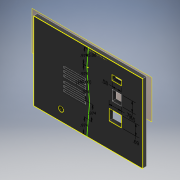
# Autodesk Inventor part: compnent box front
Saved by Autodesk Inventor 2021 (Build 250183000, 183)
## iProperties
Created: 2023-01-12
Part Number: compnent box front
Material: Generic
Document SubType Name: Modeling
Designer: boyle
Density: 1 g/cm^3
Appearance: Default
Author: boyle
Autodesk Inventor part; units mm, degrees
ref_plane "YZ Plane" through (0, 0, 0) normal (1, 0, 0) x (0, 1, 0)
ref_plane "XZ Plane" through (0, 0, 0) normal (0, 1, 0) x (-1, 0, 0)
ref_plane "XY Plane" through (0, 0, 0) normal (0, 0, 1) x (1, 0, 0)
ref_plane "Work Plane1" through (0, 0, 0) normal (0, 0, 1) x (1, 0, 0)
sketch "Sketch1" plane through (0, 0, 0) normal (0, 0, 1) x (1, 0, 0)
  line L0 (88.9, -98.425) -> (-88.9, -98.425)
  line L1 (-88.9, -98.425) -> (-88.9, -28.575)
  line L2 (-88.9, -28.575) -> (-88.9, 28.575)
  line L3 (-88.9, 28.575) -> (-85.09, 28.575)
  line L4 (88.9, 28.575) -> (88.9, -28.575)
  line L5 (85.09, 28.575) -> (88.9, 28.575)
  line L6 (88.9, -28.575) -> (88.9, -98.425)
  line L7 (-88.9, 28.575) -> (88.9, 28.575)
  line L8 (88.9, 28.575) -> (88.9, -98.425)
  line L9 (88.9, -98.425) -> (-88.9, -98.425)
  line L10 (-88.9, -98.425) -> (-88.9, 28.575)
  point P0 (0, 0)
extrude "Extrusion1" add sketch "Sketch1" along normal blind 6.35
sketch "Sketch2" plane through (0, 0, 6.35) normal (0, 0, 1) x (1, 0, 0)
  line L0 (-88.9, -98.425) -> (88.9, -98.425) projected
  line L1 (-88.9, -98.425) -> (-88.9, -28.575)
  line L2 (-88.9, 28.575) -> (-88.9, -98.425) projected
  line L3 (88.9, -98.425) -> (88.9, 28.575) projected
  circle A0 centre (-44.45, -80.9625) radius 3.937
  line L4 (-88.9, 28.575) -> (88.9, 28.575)
  line L5 (88.9, 28.575) -> (88.9, -28.575)
  line L6 (-88.9, -28.575) -> (-88.9, 28.575)
  line L7 (88.9, 28.575) -> (-88.9, 28.575) projected
  line L8 (-66.675, -80.9625) -> (-44.45, -80.9625)
  line L9 (38.7824, 9.525) -> (54.0224, 9.525)
  line L10 (54.0224, 9.525) -> (54.0224, 1.397)
  line L11 (54.0224, 1.397) -> (38.7824, 1.397)
  line L12 (38.7824, 1.397) -> (38.7824, 9.525)
  line L13 (38.7824, 9.525) -> (54.0224, 1.397) construction
  line L14 (54.0224, 9.525) -> (38.7824, 1.397) construction
  line L15 (34.2724, -40.503) -> (54.0224, -40.503)
  line L16 (54.0224, -40.503) -> (54.0224, -58.103)
  line L17 (54.0224, -58.103) -> (34.2724, -58.103)
  line L18 (34.2724, -58.103) -> (34.2724, -40.503)
  line L19 (34.2724, -40.503) -> (54.0224, -58.103) construction
  line L20 (54.0224, -40.503) -> (34.2724, -58.103) construction
  line L21 (39.3724, -11.303) -> (54.0224, -11.303)
  line L22 (54.0224, -11.303) -> (54.0224, -27.803)
  line L23 (39.3724, -27.803) -> (39.3724, -11.303)
  line L24 (39.3724, -11.303) -> (54.0224, -27.803) construction
  line L25 (54.0224, -11.303) -> (39.3724, -27.803) construction
  line L26 (-39.6628, -17.9021) -> (-3.6628, -17.9021)
  line L27 (-3.6628, -17.9021) -> (-3.6628, -53.9021)
  line L28 (-3.6628, -53.9021) -> (-39.6628, -53.9021)
  line L29 (-39.6628, -17.9021) -> (-3.6628, -53.9021) construction
  line L30 (-3.6628, -17.9021) -> (-39.6628, -53.9021) construction
  line L31 (-39.6628, -17.9021) -> (-39.6628, -53.9021)
  line L32 (-21.6628, -17.9021) -> (-21.6628, -20.9021)
  line L33 (-21.6628, -20.9021) -> (-39.6628, -20.9021)
  line L34 (-21.6628, -20.9021) -> (-3.6628, -20.9021)
  line L35 (-21.6628, -20.9021) -> (-21.6628, -23.9021)
  line L36 (-21.6628, -23.9021) -> (-39.6628, -23.9021)
  line L37 (-21.6628, -23.9021) -> (-3.6628, -23.9021)
  line L38 (-21.6628, -23.9021) -> (-21.6628, -26.9021)
  line L39 (-21.6628, -26.9021) -> (-39.6628, -26.9021)
  line L40 (-21.6628, -26.9021) -> (-3.6628, -26.9021)
  line L41 (-21.6628, -26.9021) -> (-21.6628, -29.9021)
  line L42 (-21.6628, -29.9021) -> (-39.6628, -29.9021)
  line L43 (-21.6628, -29.9021) -> (-3.6628, -29.9021)
  line L44 (-21.6628, -29.9021) -> (-21.6628, -32.9021)
  line L45 (-21.6628, -32.9021) -> (-39.6628, -32.9021)
  line L46 (-21.6628, -32.9021) -> (-3.6628, -32.9021)
  line L47 (-21.6628, -32.9021) -> (-21.6628, -35.9021)
  line L48 (-21.6628, -35.9021) -> (-39.6628, -35.9021)
  line L49 (-21.6628, -35.9021) -> (-3.6628, -35.9021)
  line L50 (-21.6628, -35.9021) -> (-21.6628, -38.9021)
  line L51 (-21.6628, -38.9021) -> (-39.6628, -38.9021)
  line L52 (-21.6628, -38.9021) -> (-3.6628, -38.9021)
  line L53 (-21.6628, -38.9021) -> (-21.6628, -41.9021)
  line L54 (-21.6628, -41.9021) -> (-39.6628, -41.9021)
  line L55 (-21.6628, -41.9021) -> (-3.6628, -41.9021)
  line L56 (-21.6628, -41.9021) -> (-21.6628, -44.9021)
  line L57 (-21.6628, -44.9021) -> (-39.6628, -44.9021)
  line L58 (-21.6628, -44.9021) -> (-3.6628, -44.9021)
  line L59 (-21.6628, -44.9021) -> (-21.6628, -47.9021)
  line L60 (-21.6628, -47.9021) -> (-39.6628, -47.9021)
  line L61 (-21.6628, -47.9021) -> (-3.6628, -47.9021)
  line L62 (-21.6628, -47.9021) -> (-21.6628, -50.9021)
  line L63 (-21.6628, -50.9021) -> (-39.6628, -50.9021)
  line L64 (-21.6628, -50.9021) -> (-3.6628, -50.9021)
  line L65 (-21.6628, -50.9021) -> (-21.6628, -53.9021)
  line L66 (-21.6628, -53.9021) -> (-39.6628, -53.9021)
  line L67 (-21.6628, -53.9021) -> (-3.6628, -53.9021)
  line L68 (39.3724, -27.803) -> (54.0224, -27.803)
  line L69 (54.0224, 28.575) -> (54.0224, 9.525)
  line L70 (54.0224, 1.397) -> (54.0224, -11.303)
  line L71 (54.0224, -27.803) -> (54.0224, -40.503)
  point P0 (44.1474, -49.303)
  point P1 (46.6974, -19.553)
  point P2 (-3.6628, -41.9021)
  point P3 (-3.6628, -38.9021)
  point P4 (-3.6628, -47.9021)
  point P5 (-3.6628, -44.9021)
  point P6 (-3.6628, -50.9021)
  point P7 (-3.6628, -32.9021)
  point P8 (-3.6628, -29.9021)
  point P9 (-3.6628, -26.9021)
  point P10 (-3.6628, -23.9021)
  dimension "d2" = 69.85
  dimension "d5" = 7.874
  dimension "d8" = 15.24
  dimension "d9" = 8.128
  dimension "d10" = 16.5
  dimension "d11" = 14.65
  dimension "d12" = 19.75
  dimension "d13" = 17.6
  dimension "d34" = 36
  dimension "d35" = 36
  dimension "d39" = 3
  dimension "d40" = 3
  dimension "d41" = 3
  dimension "d42" = 3
  dimension "d43" = 3
  dimension "d44" = 3
  dimension "d45" = 3
  dimension "d46" = 3
  dimension "d47" = 3
  dimension "d48" = 3
  dimension "d49" = 3
  dimension "d50" = 3
  dimension "d51" = 19.05
  dimension "d52" = 12.7
  dimension "d53" = 12.7
  constraints: 136 end point, 14 vertical, 7 parallel, 7 perpendicular, 6 horizontal, 5 midpoint, 5 point on line, 1 centre point
  measures "d2" distance of L0.start L1.end
  measures "d5" diameter of A0
  measures "d8" distance of L9.start L9.end
  measures "d9" distance of L9.end L10.end
  measures "d10" distance of L22.end L21.end
  measures "d11" distance of L21.start L21.end
  measures "d12" distance of L15.start L15.end
  measures "d13" distance of L15.end L16.end
  measures "d34" distance of L27.end L28.end
  measures "d35" distance of L26.end L27.end
  measures "d39" distance of L32.start L32.end
  measures "d40" distance of L35.start L35.end
  measures "d41" distance of L38.start L38.end
  measures "d42" distance of L41.start L41.end
  measures "d43" distance of L44.start L44.end
  measures "d44" distance of L47.start L47.end
  measures "d45" distance of L50.start L50.end
  measures "d46" distance of L53.start L53.end
  measures "d47" distance of L56.start L56.end
  measures "d48" distance of L59.start L59.end
  measures "d49" distance of L62.start L62.end
  measures "d50" distance of L65.start L65.end
  measures "d51" distance of L69.start L69.end
  measures "d52" distance of L10.end L70.end
  measures "d53" distance of L24.end L71.end
extrude "Extrusion2" cut sketch "Sketch2" against normal through all contours A0 | L9 L10 L11 L12 | L15 L16 L17 L18 | L21 L22 L68 L23 | L26 L32 L33 L31 | L26 L27 L34 L32 | L36 L38 L39 L31 | L37 L27 L40 L38 | L42 L44 L45 L31 | L43 L27 L46 L44 | L51 L53 L54 L31 | L52 L27 L55 L53 | L57 L59 L60 L31 | L58 L27 L61 L59 | L63 L65 L28 L31 | L64 L27 L28 L65
sketch "Sketch3" plane through (0, 0, 6.35) normal (0, 0, 1) x (1, 0, 0)
  line L0 (88.9, 28.575) -> (-88.9, 28.575) projected
  line L1 (-88.9, -98.425) -> (88.9, -98.425) projected
  line L2 (-88.9, -98.425) -> (88.9, -98.425) projected
  line L3 (0, 25.29) -> (30.48, 25.29) construction
  line L4 (0, 25.29) -> (-2.1566, 0.6394)
  line L5 (0, 25.29) -> (24.7447, 25.29) construction
  line L6 (-2.1566, 0.6394) -> (0, -24.0111)
  line L7 (0, -24.0111) -> (2.1566, -48.6616)
  line L8 (2.1566, -48.6616) -> (0, -73.3121)
  line L9 (0, -73.3121) -> (-2.1566, -97.9626)
  line L10 (0, 25.29) -> (0, 28.575)
  line L11 (-2.1566, -97.9626) -> (-2.1566, -98.425)
  line L12 (-88.9, 28.575) -> (-88.9, -98.425) projected
  line L13 (54.0224, 1.397) -> (38.7824, 1.397) projected
  line L14 (38.7824, 1.397) -> (38.7824, 9.525) projected
  line L15 (38.7824, 9.525) -> (54.0224, 9.525) projected
  line L16 (54.0224, 9.525) -> (54.0224, 1.397) projected
  line L17 (54.0224, -40.503) -> (54.0224, -58.103) projected
  line L18 (54.0224, -58.103) -> (34.2724, -58.103) projected
  line L19 (34.2724, -58.103) -> (34.2724, -40.503) projected
  line L20 (34.2724, -40.503) -> (54.0224, -40.503) projected
  circle A0 centre (-44.45, -80.9625) radius 3.937 projected
  line L21 (88.9, 28.575) -> (-88.9, 28.575) projected
  line L22 (-88.9, 28.575) -> (-88.9, -98.425) projected
  line L23 (-88.9, -98.425) -> (88.9, -98.425) projected
  line L24 (88.9, -98.425) -> (88.9, 28.575) projected
  point P0 (0, 0)
  dimension "d21" = 24.7447
  dimension "d22" = 95
  dimension "d23" = 24.7447
  dimension "d24" = 24.7447
  dimension "d25" = 180
  dimension "d26" = 24.7447
  dimension "d27" = 24.7447
  constraints: 18 end point, 2 horizontal, 2 point on line, 1 collinear, 1 equal length, 1 midpoint, 1 perpendicular
  measures "d21" distance of L3.start L4.end
  measures "d22" angle of L4 L5
  measures "d23" distance of L4.end L6.end
  measures "d24" distance of L6.end L7.end
  measures "d25" angle of L7 L6
  measures "d26" distance of L7.end L8.end
  measures "d27" distance of L8.end L9.end
body "Solid1"
